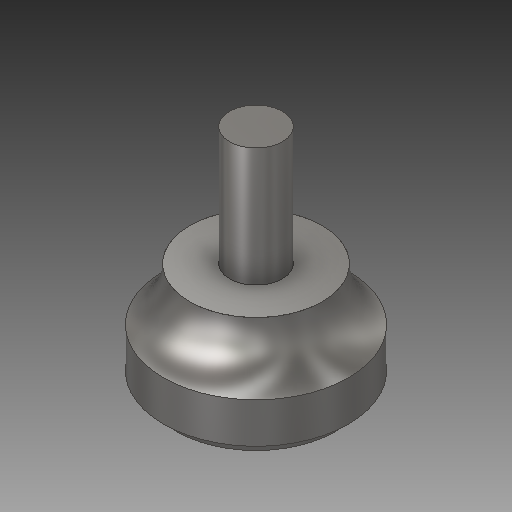
# Autodesk Inventor part: Rack Pad
Saved by Autodesk Inventor 2018 (Build 220112000, 112)
## iProperties
Created: 2017-12-21
Part Number: Rack Pad
Material: Stainless Steel
Document SubType Name: Modeling
Designer: 232963
Density: 8 g/cm^3
Appearance: Semi-Polished
Mass: 35.4776 g
Surface Area: 16.6674 cm^2
Volume: 4.43471 cm^3
Author: 232963
Autodesk Inventor part; units mm, degrees
ref_plane "YZ Plane" through (0, 0, 0) normal (1, 0, 0) x (0, 1, 0)
ref_plane "XZ Plane" through (0, 0, 0) normal (0, 1, 0) x (-1, 0, 0)
ref_plane "XY Plane" through (0, 0, 0) normal (0, 0, 1) x (1, 0, 0)
sketch "Sketch1" plane through (0, 0, 0) normal (0, 0, 1) x (1, 0, 0)
  line L0 (0, 0) -> (11.1125, 0)
  line L1 (11.1125, 0) -> (11.1125, 6.35)
  line L2 (3.175, 26.9748) -> (0, 26.9748)
  line L3 (0, 26.9748) -> (0, 0)
  line L4 (3.175, 26.9748) -> (3.175, 12.7)
  line L5 (3.175, 12.7) -> (7.9502, 12.7)
  line L6 (7.9502, 12.7) -> (7.9502, 6.35)
  line L7 (7.9502, 6.35) -> (11.1125, 6.35)
  dimension "d2" = 3.175
  dimension "d3" = 7.9502
  constraints: 16 end point, 5 perpendicular, 2 parallel, 1 horizontal
  measures "d2" distance between parallel lines of L3 L4
  measures "d3" distance between parallel lines of L3 L6
revolve "Revolution1" add sketch "Sketch1" angle 360 about axis through (0, 26.9748, 0) along (0, -1, 0)
fillet "Fillet1" radius 7.9248 1 edges at (-7.9502, 6.35, 0)
chamfer "Chamfer1" distance 1.524 angle 45 1 edges at (-11.1125, 0, 0)
body "Solid1"
